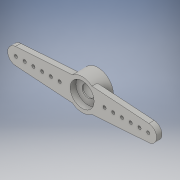
# Autodesk Inventor part: 1 Way MicroServo Attachment
Saved by Autodesk Inventor 2016 (Build 200138000, 138)
## iProperties
Created: 2016-02-12
Part Number: 1 Way MicroServo Attachment
Material: Generic
Document SubType Name: Modeling
Designer: RoksBot
Density: 1 g/cm^3
Appearance: Default
Author: RoksBot
Autodesk Inventor part; units mm, degrees
ref_plane "YZ Plane" through (0, 0, 0) normal (1, 0, 0) x (0, 1, 0)
ref_plane "XZ Plane" through (0, 0, 0) normal (0, 1, 0) x (-1, 0, 0)
ref_plane "XY Plane" through (0, 0, 0) normal (0, 0, 1) x (1, 0, 0)
sketch "Sketch1" plane through (0, 0, 0) normal (0, 0, 1) x (1, 0, 0)
  circle A0 centre (0, 0) radius 3.4036
  circle A1 centre (-14.4145, 0) radius 1.8161
  circle A2 centre (14.4145, 0) radius 1.8161
  line L0 (0, 0) -> (0, 12.9246) construction
  line L1 (-14.5375, 1.8119) -> (-2.1305, 2.6543)
  line L2 (2.1305, 2.6543) -> (14.5375, 1.8119)
  line L3 (14.5375, -1.8119) -> (2.1305, -2.6543)
  line L4 (-2.1305, -2.6543) -> (-14.5375, -1.8119)
  dimension "d0" = 6.8072
  dimension "d1" = 3.6322
  dimension "d2" = 32.4612
  dimension "d3" = 5.3086
  constraints: 10 end point, 8 point on circle, 4 tangent, 3 centre point, 3 equal length, 1 coincident, 1 horizontal alignment, 1 vertical, 1 other
  measures "d0" diameter of A0
  measures "d1" diameter of A1
  measures "d3" distance of L4.start L1.end
extrude "Extrusion1" add sketch "Sketch1" along normal blind 1.1684
sketch "Sketch2" plane through (0, 0, 0) normal (0, 0, -1) x (-1, 0, 0)
  arc A0 (14.5375, -1.8119) -> (14.5375, 1.8119) centre (14.4145, 0) ccw projected
  line L0 (2.1305, 2.6543) -> (14.5375, 1.8119) projected
  arc A1 (2.1305, 2.6543) -> (-2.1305, 2.6543) centre (0, 0) ccw projected
  line L1 (-14.5375, 1.8119) -> (-2.1305, 2.6543) projected
  arc A2 (-14.5375, 1.8119) -> (-14.5375, -1.8119) centre (-14.4145, 0) ccw projected
  line L2 (-2.1305, -2.6543) -> (-14.5375, -1.8119) projected
  arc A3 (-2.1305, -2.6543) -> (2.1305, -2.6543) centre (0, 0) ccw projected
  line L3 (14.5375, -1.8119) -> (2.1305, -2.6543) projected
  circle A4 centre (0, 0) radius 3.4036
  constraints: 1 coincident, 3 other
extrude "Extrusion2" add sketch "Sketch2" along normal blind 2.2606 contours A3 A4 A1
sketch "Sketch3" plane through (0, 0, -2.2606) normal (0, 0, -1) x (-1, 0, 0)
  circle A0 centre (0, 0) radius 2.2733
  dimension "d8" = 4.5466
  constraints: 1 centre point, 1 coincident
  measures "d8" diameter of A0
extrude "Extrusion3" cut sketch "Sketch3" against normal blind 1.905
sketch "Sketch4" plane through (0, 0, 1.1684) normal (0, 0, 1) x (1, 0, 0)
  circle A0 centre (0, 0) radius 2.6162
  dimension "d11" = 5.2324
  constraints: 1 centre point, 1 coincident
  measures "d11" diameter of A0
extrude "Extrusion4" cut sketch "Sketch4" against normal blind 1.27
sketch "Sketch5" plane through (0, 0, -0.1016) normal (0, 0, 1) x (1, 0, 0)
  circle A0 centre (0, 0) radius 1.2954
  dimension "d14" = 2.5908
  constraints: 1 centre point, 1 coincident
  measures "d14" diameter of A0
extrude "Extrusion5" cut sketch "Sketch5" against normal blind 1.27
sketch "Sketch6" plane through (0, 0, 1.1684) normal (0, 0, 1) x (1, 0, 0)
  arc A0 (-14.5375, 1.8119) -> (-14.5375, -1.8119) centre (-14.4145, 0) ccw projected
  circle A1 centre (-14.4145, 0) radius 0.3429
  point P0 (0, 0)
  dimension "d17" = 0.6858
  constraints: 1 centre point, 1 coincident
  measures "d17" diameter of A1
extrude "Extrusion6" cut sketch "Sketch6" against normal through all
pattern_linear "Rectangular Pattern1" count 6 spacing 1.905 along (1, 0, 0) of "Extrusion6"
mirror "Mirror1" about plane through (0, 0, 0) normal (1, 0, 0) of "Extrusion6", "Rectangular Pattern1"
body "Solid1"
